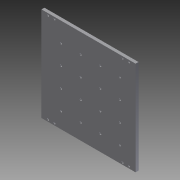
# Autodesk Inventor part: baseplate
Saved by Autodesk Inventor 2012 (Build 160160000, 160)
## iProperties
Created: 2011-09-20
Part Number: baseplate
Material: Default
Document SubType Name: Modeling
Designer: shane
Density: 1 g/cm^3
Author: shane
Autodesk Inventor part; units mm, degrees
ref_plane "YZ Plane" through (0, 0, 0) normal (1, 0, 0) x (0, 1, 0)
ref_plane "XZ Plane" through (0, 0, 0) normal (0, 1, 0) x (-1, 0, 0)
ref_plane "XY Plane" through (0, 0, 0) normal (0, 0, 1) x (1, 0, 0)
sketch "Sketch1" plane through (0, 0, 0) normal (0, 0, 1) x (1, 0, 0)
  line L0 (0, 304.8) -> (304.8, 304.8)
  line L1 (304.8, 304.8) -> (304.8, 0)
  line L2 (304.8, 0) -> (0, 0)
  line L3 (0, 0) -> (0, 304.8)
  dimension "d0" = 304.8
  dimension "d1" = 304.8
  constraints: 8 end point, 2 parallel, 1 horizontal, 1 perpendicular
  measures "d0" distance of L2.end L0.start
  measures "d1" distance of L1.end L2.end
extrude "Extrusion1" add sketch "Sketch1" along normal blind 9.525
hole "Hole1" at (21.336, 298.45, 9.525) direction (0, 0, -1) diameter 6.35 end through all
hole "Hole2" at (42.164, 298.45, 9.525) direction (0, 0, -1) diameter 6.35 end through all
hole "Hole3" at (262.636, 298.45, 9.525) direction (0, 0, -1) diameter 6.35 end through all
hole "Hole4" at (283.464, 298.45, 9.525) direction (0, 0, -1) diameter 6.35 end through all
hole "Hole5" at (21.336, 6.35, 9.525) direction (0, 0, -1) diameter 6.35 end through all
hole "Hole6" at (42.164, 6.35, 9.525) direction (0, 0, -1) diameter 6.35 end through all
hole "Hole7" at (262.636, 6.35, 9.525) direction (0, 0, -1) diameter 6.35 end through all
hole "Hole8" at (283.464, 6.35, 9.525) direction (0, 0, -1) diameter 6.35 end through all
hole "Hole9" at (63.5, 241.3, 9.525) direction (0, 0, -1) diameter 6.35 end through all
pattern_linear "Rectangular Pattern1" count 4 spacing 63.5 along (1, 0, 0) count 4 spacing 63.5 along (0, -1, 0) of "Hole9"
body "Solid1"
